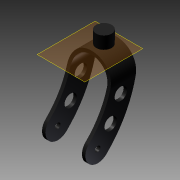
# Autodesk Inventor part: caster
Saved by Autodesk Inventor 2012 (Build 160160000, 160)
## iProperties
Created: 2012-03-07
Part Number: caster
Material: Default
Document SubType Name: Modeling
Designer: esv
Density: 1 g/cm^3
Author: esv
Autodesk Inventor part; units mm, degrees
ref_plane "YZ Plane" through (0, 0, 0) normal (1, 0, 0) x (0, 1, 0)
ref_plane "XY Plane" through (0, 0, 0) normal (0, 0, 1) x (1, 0, 0)
sketch "Sketch1" plane through (0, 0, 0) normal (0, 0, 1) x (1, 0, 0)
  line L0 (-37.4396, -25.4) -> (-44.45, -25.4)
  line L1 (-44.45, -25.4) -> (-44.45, 92.075)
  line L2 (-44.45, 92.075) -> (-37.4396, 92.075)
  line L3 (-37.4396, 92.075) -> (-37.4396, -25.4)
  line L4 (44.45, -25.4) -> (37.4396, -25.4)
  line L5 (37.4396, -25.4) -> (37.4396, 92.075)
  line L6 (37.4396, 92.075) -> (44.45, 92.075)
  line L7 (44.45, 92.075) -> (44.45, -25.4)
  arc A0 (37.4396, 92.075) -> (-37.4396, 92.075) centre (0, 92.075) ccw
  arc A1 (44.45, 92.075) -> (-44.45, 92.075) centre (0, 92.075) ccw
  line L8 (0, 136.525) -> (-29.2204, 136.525)
  point P0 (0, 0)
  dimension "d0" = 161.925
  dimension "d1" = 7.0104
  dimension "d2" = 88.9
  dimension "d3" = 25.4
  constraints: 18 end point, 5 point on circle, 4 parallel, 4 tangent, 3 perpendicular, 2 centre point, 2 horizontal, 1 collinear, 1 point on line, 1 vertical alignment
  measures "d0" distance between parallel lines of L8 L0
  measures "d1" distance between parallel lines of L1 L3
  measures "d2" distance between parallel lines of L7 L1
  measures "d3" distance from line of point (0, 0) L0
extrude "Extrusion1" add sketch "Sketch1" along normal blind 107.95
sketch "Sketch2" plane through (44.45, -25.4, 0) normal (1, 0, 0) x (0, 0, -1)
  line L0 (-107.95, 117.475) -> (-107.95, 0) projected
  line L1 (0, 0) -> (-107.95, 0) projected
  line L2 (0, 0) -> (0, 117.475) projected
  line L3 (0, 117.475) -> (-107.95, 117.475) projected
  circle A0 centre (-82.55, 25.4) radius 25.4
  arc A1 (-64.7244, 7.3056) -> (0, 161.925) centre (-217.0465, 161.925) ccw
  arc A2 (-100.3756, 43.4944) -> (-50.8, 161.925) centre (-217.0465, 161.925) ccw
  line L4 (0, 161.925) -> (-50.8, 161.925)
  circle A3 centre (-56.1006, 57.0868) radius 12.7
  circle A4 centre (-35.1643, 99.8631) radius 12.7
  arc A5 (-82.55, 25.4) -> (-25.4, 161.925) centre (-210.7426, 159.2862) ccw
  point P0 (0, 25.4)
  dimension "d7" = 50.8
  dimension "d8" = 161.925
  dimension "d9" = 25.4
  dimension "d10" = 47.625
  dimension "d11" = 41.275
  dimension "d12" = 185.3614
  constraints: 10 point on circle, 6 centre point, 5 tangent, 2 end point, 1 concentric, 1 equal radius, 1 midpoint, 1 parallel, 1 vertical alignment
  measures "d7" distance of L4.start L4.end
  measures "d8" distance between parallel lines of L1 L4
  measures "d9" diameter of A4
  measures "d10" distance of A4.centre A3.centre
  measures "d11" distance of A3.centre A0.centre
  measures "d12" radius of A5
extrude "Extrusion2" cut sketch "Sketch2" against normal through all contours A0 | A2 L4 A5 L3 | L3 A5 A4 A3 A0 A2 | A5 L4 A1 L3 | L3 A1 A0 A5 A3 A4 keep common part
hole "Hole1" at (44.45, 0, 82.55) direction (-1, 0, 0) diameter 10.9982 end through all clearance for "Flat Head Machine Screw" size "M10" standard "Ansi Metric M Profile"
ref_plane "Work Plane1" through (0, 136.525, 0) normal (0, 1, 0) x (-1, 0, 0)
sketch "Sketch3" plane through (0, 136.525, 0) normal (0, 1, 0) x (-1, 0, 0)
  circle A0 centre (0, 25.4) radius 15.875
  point P0 (0, 0)
  dimension "d24" = 25.4
  dimension "d25" = 31.75
  constraints: 1 centre point, 1 vertical alignment
  measures "d24" distance of A0.centre point (0, 0)
  measures "d25" diameter of A0
extrude "Extrusion3" add sketch "Sketch3" along normal blind 25.4
body "Solid1"
